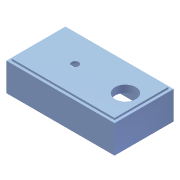
# Autodesk Inventor part: Casing
Saved by Autodesk Inventor 2012 (Build 160160000, 160)
## iProperties
Created: 2017-01-26
Part Number: Casing
Material: Default
Document SubType Name: Modeling
Designer: omaro
Density: 1 g/cm^3
Author: omaro
Autodesk Inventor part; units mm, degrees
ref_plane "YZ Plane" through (0, 0, 0) normal (1, 0, 0) x (0, 1, 0)
ref_plane "XZ Plane" through (0, 0, 0) normal (0, 1, 0) x (-1, 0, 0)
ref_plane "XY Plane" through (0, 0, 0) normal (0, 0, 1) x (1, 0, 0)
sketch "Sketch1" plane through (0, 0, 0) normal (0, 0, 1) x (1, 0, 0)
  line L0 (-60.6, 33.1) -> (60.6, 33.1)
  line L1 (60.6, 33.1) -> (60.6, -33.1)
  line L2 (60.6, -33.1) -> (-60.6, -33.1)
  line L3 (-60.6, -33.1) -> (-60.6, 33.1)
  line L4 (57.7, 30.2) -> (-57.7, 30.2)
  line L5 (-57.7, 30.2) -> (-57.7, -30.2)
  line L6 (-57.7, -30.2) -> (57.7, -30.2)
  line L7 (57.7, -30.2) -> (57.7, 30.2)
  point P0 (0, 0)
  dimension "d0" = 121.2
  dimension "d1" = 66.2
  dimension "d2" = 60.6
  dimension "d3" = 33.1
  dimension "d4" = 2.9
  constraints: 16 end point, 4 parallel, 2 perpendicular, 1 horizontal, 3 other
  measures "d0" distance of L0.start L0.end
  measures "d1" distance of L2.end L0.start
  measures "d2" distance from line of L3 point (0, 0)
  measures "d3" distance from line of L2 point (0, 0)
  measures "d4" distance between parallel lines of L0 L4
extrude "Extrusion1" add sketch "Sketch1" along normal mid plane 31.5
sketch "Sketch2" plane through (0, 0, 15.75) normal (0, 0, 1) x (1, 0, 0)
  line L0 (-57.7, 30.2) -> (57.7, 30.2)
  line L1 (57.7, 30.2) -> (57.7, -30.2)
  line L2 (57.7, -30.2) -> (-57.7, -30.2)
  line L3 (-57.7, -30.2) -> (-57.7, 30.2)
  point P0 (0, 0)
  constraints: 8 end point, 2 parallel, 1 horizontal, 1 perpendicular
extrude "Extrusion2" add sketch "Sketch2" along normal blind 2.1
sketch "Sketch3" plane through (0, 0, 15.75) normal (0, 0, -1) x (-1, 0, 0)
  line L0 (57.7, -30.2) -> (57.7, 30.2) projected
  line L1 (57.7, 30.2) -> (-57.7, 30.2) projected
  line L2 (-57.7, 30.2) -> (-57.7, -30.2) projected
  line L3 (-57.7, -30.2) -> (57.7, -30.2) projected
  line L4 (-57.7, -30.2) -> (-57.7, 30.2) projected
  line L5 (57.7, -30.2) -> (57.7, 30.2) projected
  line L6 (57.7, 30.2) -> (-57.7, 30.2) projected
  line L7 (-57.7, 30.2) -> (-57.7, -30.2) projected
  line L8 (-57.7, -30.2) -> (57.7, -30.2) projected
  circle A0 centre (16.7, 0) radius 4.05
  circle A1 centre (-39.7, 0) radius 11.6414
  point P0 (0, 0)
  dimension "d9" = 8.1
  dimension "d10" = 41
  dimension "d11" = 30.2
  dimension "d12" = 30.2
  dimension "d13" = 18
  dimension "d28" = 60.4
  constraints: 2 centre point
  measures "d9" diameter of A0
  measures "d10" distance from line of L0 A0.centre
  measures "d11" distance from line of L3 A0.centre
  measures "d12" distance from line of L1 A1.centre
  measures "d13" distance from line of L2 A1.centre
  measures "d28" distance of L0.start L0.end
extrude "Extrusion3" cut sketch "Sketch3" against normal through all contours A0 | A1
sketch "Sketch4" plane through (0, 0, 15.75) normal (0, 0, -1) x (-1, 0, 0)
  circle A0 centre (-39.7, 0) radius 11.6414 projected
  circle A1 centre (-39.7, 0) radius 13.1414
  point P0 (0, 0)
  dimension "d16" = 23.2828
  dimension "d17" = 26.2828
  constraints: 1 centre point, 1 coincident
  measures "d16" diameter of A0
  measures "d17" diameter of A1
extrude "Extrusion4" add sketch "Sketch4" along normal blind 6
sketch "Sketch5" plane through (0, 0, 15.75) normal (0, 0, -1) x (-1, 0, 0)
  circle A0 centre (-39.7, 0) radius 13.1414 projected
  circle A1 centre (-7.9, 0) radius 4.55
  circle A2 centre (16.7, 0) radius 4.05 projected
  line L0 (57.7, -30.2) -> (57.7, 30.2) projected
  point P0 (0, 0)
  dimension "d20" = 9.1
  dimension "d21" = 31.8
  dimension "d22" = 0
  dimension "d29" = 24.6
  dimension "d30" = 65.6
  dimension "d31" = 8.1
  dimension "d32" = 41
  constraints: 1 centre point
  measures "d20" diameter of A1
  measures "d21" distance of A0.centre A1.centre
  measures "d22" vertical distance of A0.centre A1.centre
  measures "d29" distance of A2.centre A1.centre
  measures "d30" distance from line of L0 A1.centre
  measures "d31" diameter of A2
  measures "d32" distance from line of L0 A2.centre
extrude "Extrusion5" add sketch "Sketch5" along normal blind 2.4 contours A1
sketch "Sketch6" plane through (7.9, 0, 13.35) normal (0, 0, -1) x (-1, 0, 0)
  circle A0 centre (0, 0) radius 4.55 projected
  circle A1 centre (0, 0) radius 2.55
  point P0 (7.9, 0)
  dimension "d25" = 5.1
  constraints: 1 centre point, 1 coincident
  measures "d25" diameter of A1
extrude "Extrusion6" add sketch "Sketch6" along normal blind 29 contours A1
sketch "Sketch7" plane through (0, 0, 15.75) normal (0, 0, -1) x (-1, 0, 0)
  circle A0 centre (-7.9, 0) radius 4.55 projected
  circle A1 centre (16.7, 0) radius 4.05 projected
  circle A2 centre (14.1, 14.05) radius 10
  point P0 (0, 0)
  dimension "d33" = 14.05
  dimension "d34" = 20
  dimension "d36" = 22
  dimension "d37" = 8.1
  constraints: 1 centre point
  measures "d33" vertical distance of A1.centre A2.centre
  measures "d34" diameter of A2
  measures "d36" horizontal distance of A0.centre A2.centre
  measures "d37" diameter of A1
extrude "Extrusion7" add sketch "Sketch7" along normal blind 12 contours A2
equation "\"d2\" = 0.5 * d0"
equation "\"d3\" = 0.5 * d1"
equation "\"d11\" = 0.5 * d28"
equation "\"d12\" = d11"
equation "\"d33\" = 0.5 * d37 + 0.5 * d34"
body "Solid1"
